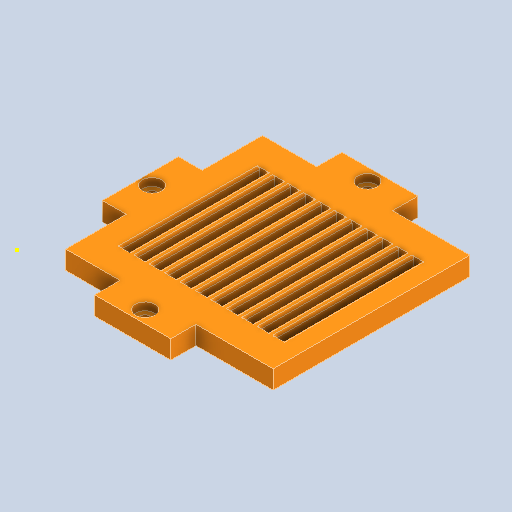
# Autodesk Inventor part: Tapa - Caja para Electrónica
Saved by Autodesk Inventor 2026 (Build 300175050, 175E)
## iProperties
Created: 2026-02-11
Part Number: Tapa - Caja para Electrónica
Material: Genérico
Document SubType Name: Modeling
Designer: bello
Density: 1 g/cm^3
Appearance: Naranja
Author: bello
Autodesk Inventor part; units mm, degrees
ref_plane "YZ Plane" through (0, 0, 0) normal (1, 0, 0) x (0, 1, 0)
ref_plane "XZ Plane" through (0, 0, 0) normal (0, 1, 0) x (-1, 0, 0)
ref_plane "XY Plane" through (0, 0, 0) normal (0, 0, 1) x (1, 0, 0)
sketch "Boceto1" plane through (0, 0, 0) normal (0, 1, 0) x (-1, 0, 0)
  line L0 (0, 0) -> (-75, 0)
  line L1 (-75, 0) -> (-75, -80)
  line L2 (-75, -80) -> (0, -80)
  line L3 (0, -80) -> (0, 0)
  dimension "d0" = 80
  dimension "d1" = 75
  constraints: 8 end point, 2 parallel, 1 horizontal, 1 perpendicular
  measures "d0" distance of L2.end L0.start
  measures "d1" distance of L1.end L2.end
extrude "Extrusión1" add sketch "Boceto1" along normal blind 6
sketch "Boceto2" plane through (0, 6, 0) normal (0, 1, 0) x (1, 0, 0)
  line L0 (0, 0) -> (75, 0) projected
  line L1 (25, 0) -> (25, 8)
  line L2 (25, 8) -> (7.5, 8)
  line L3 (7.5, 8) -> (7.5, 27.5)
  line L4 (7.5, 27.5) -> (0, 27.5)
  line L5 (0, 27.5) -> (0, 40)
  line L6 (25, 0) -> (50, 0)
  line L7 (50, 0) -> (50, 8)
  line L8 (50, 8) -> (75, 8)
  line L9 (75, 0) -> (75, 80) projected
  line L10 (-21.9373, 40) -> (100.0778, 40)
  line L11 (25, 0) -> (50, 0)
  line L12 (25, 80) -> (25, 72)
  line L13 (25, 72) -> (7.5, 72)
  line L14 (7.5, 72) -> (7.5, 52.5)
  line L15 (7.5, 52.5) -> (0, 52.5)
  line L16 (0, 52.5) -> (0, 40)
  line L17 (50, 80) -> (50, 72)
  line L18 (50, 72) -> (75, 72)
  line L19 (25, 80) -> (50, 80)
  line L20 (75, 80) -> (0, 80) projected
  line L21 (0, 80) -> (0, 0) projected
  dimension "d4" = 12.5
  dimension "d7" = 8
  dimension "d8" = 25
  dimension "d9" = 25
  dimension "d10" = 12.5
  dimension "d11" = 27.5
  dimension "d12" = 27.5
  dimension "d13" = 8
  dimension "d14" = 8
  dimension "d15" = 8
  dimension "d16" = 7.5
  dimension "d17" = 25
  dimension "d18" = 25
  dimension "d19" = 25
  dimension "d20" = 25
  constraints: 36 end point, 8 symmetric about line, 4 perpendicular, 3 point on line, 2 horizontal, 1 collinear, 1 vertical
  measures "d4" distance of L4.end L5.end
  measures "d7" distance between parallel lines of L0 L2
  measures "d8" distance of L1.start L6.end
  measures "d9" distance of L7.end L8.end
  measures "d10" distance of L16.start L5.end
  measures "d11" distance between parallel lines of L20 L15
  measures "d12" distance between parallel lines of L0 L4
  measures "d13" distance between parallel lines of L20 L13
  measures "d14" distance between parallel lines of L20 L18
  measures "d15" distance between parallel lines of L0 L8
  measures "d16" distance between parallel lines of L21 L14
  measures "d17" distance of L12.start L19.end
  measures "d18" distance of L17.end L18.end
  measures "d19" distance between parallel lines of L21 L12
  measures "d20" distance between parallel lines of L21 L1
extrude "Extrusión2" cut sketch "Boceto2" against normal through all contours L21 L4 L3 L2 L1 L0 | L7 L8 L9 L0 | L21 L20 L12 L13 L14 L15 | L18 L17 L20 L9
sketch "Boceto3" plane through (0, 6, 0) normal (0, 1, 0) x (1, 0, 0)
  circle A0 centre (3.75, 40) radius 1.5
  circle A1 centre (37.5, 76) radius 1.5
  circle A2 centre (37.5, 4) radius 1.5
  line L0 (7.5, 52.5) -> (0, 52.5) projected
  line L1 (0, 52.5) -> (0, 27.5) projected
  line L2 (50, 80) -> (25, 80) projected
  line L3 (25, 0) -> (50, 0) projected
  line L4 (50, 0) -> (50, 8) projected
  line L5 (50, 72) -> (50, 80) projected
  point P0 (0, 0)
  dimension "d23" = 3
  dimension "d24" = 12.5
  dimension "d25" = 3.75
  dimension "d26" = 4
  dimension "d27" = 4
  dimension "d28" = 12.5
  dimension "d29" = 12.5
  constraints: 3 centre point, 2 equal radius
  measures "d23" diameter of A0
  measures "d24" distance from line of L0 A0.centre
  measures "d25" distance from line of L1 A0.centre
  measures "d26" distance from line of L2 A1.centre
  measures "d27" distance from line of L3 A2.centre
  measures "d28" distance from line of L4 A2.centre
  measures "d29" distance from line of L5 A1.centre
extrude "Extrusión3" cut sketch "Boceto3" against normal through all
sketch "Boceto4" plane through (0, 6, 0) normal (0, 1, 0) x (1, 0, 0)
  circle A0 centre (3.75, 40) radius 1.5 projected
  circle A1 centre (3.75, 40) radius 3.1
  circle A2 centre (37.5, 4) radius 1.5 projected
  circle A3 centre (37.5, 4) radius 3.1
  circle A4 centre (37.5, 76) radius 1.5 projected
  circle A5 centre (37.5, 76) radius 3.1
  point P0 (0, 0)
  dimension "d32" = 6.2
  constraints: 3 centre point, 3 coincident, 2 equal radius
  measures "d32" diameter of A1
extrude "Extrusión4" cut sketch "Boceto4" against normal blind 2.5 contours A0 | A1 | A2 | A3 | A5
sketch "Boceto5" plane through (0, 6, 0) normal (0, 1, 0) x (1, 0, 0)
  line L0 (0, 52.5) -> (0, 27.5) projected
  line L1 (7.5, 52.5) -> (0, 52.5) projected
  line L2 (0, 52.5) -> (7.5, 52.5)
  line L3 (7.5, 52.5) -> (7.5, 52.3)
  line L4 (7.5, 52.3) -> (0, 52.3)
  line L5 (0, 52.3) -> (0, 52.5)
  line L6 (25, 80) -> (25, 72) projected
  line L7 (25, 80) -> (25.2, 80)
  line L8 (25.2, 80) -> (25.2, 71.85)
  line L9 (25.2, 71.85) -> (25, 71.85)
  line L10 (25, 71.85) -> (25, 80)
  line L11 (7.5, 72) -> (25, 72)
  line L12 (25, 72) -> (25, 71.85)
  line L13 (25, 71.85) -> (7.5, 71.85)
  line L14 (7.5, 71.85) -> (7.5, 72)
  line L15 (7.5, 52.3) -> (7.65, 52.3)
  line L16 (7.65, 52.3) -> (7.65, 72)
  line L17 (7.65, 72) -> (7.5, 72)
  line L18 (7.5, 72) -> (7.5, 52.3)
  line L19 (50, 80) -> (25, 80) projected
  line L20 (50, 80) -> (49.8, 80)
  line L21 (49.8, 80) -> (49.8, 71.85)
  line L22 (49.8, 71.85) -> (50, 71.85)
  line L23 (50, 71.85) -> (50, 80)
  line L24 (50, 71.85) -> (75, 71.85)
  line L25 (75, 71.85) -> (75, 72)
  line L26 (75, 72) -> (50, 72)
  line L27 (50, 72) -> (50, 71.85)
  line L28 (50, 8) -> (75, 8) projected
  line L29 (75, 8) -> (74.8, 8)
  line L30 (74.8, 8) -> (74.8, 72)
  line L31 (74.8, 72) -> (75, 72)
  line L32 (75, 72) -> (75, 8)
  line L33 (-2.8758, 40) -> (82.3038, 40)
  line L34 (7.5, 27.5) -> (0, 27.5)
  line L35 (0, 27.5) -> (7.5, 27.5)
  line L36 (7.5, 27.5) -> (7.5, 27.7)
  line L37 (7.5, 27.7) -> (0, 27.7)
  line L38 (0, 27.7) -> (0, 27.5)
  line L39 (25, 0) -> (25, 8)
  line L40 (25, 0) -> (25.2, 0)
  line L41 (25.2, 0) -> (25.2, 8.15)
  line L42 (25.2, 8.15) -> (25, 8.15)
  line L43 (25, 8.15) -> (25, 0)
  line L44 (7.5, 8) -> (25, 8)
  line L45 (25, 8) -> (25, 8.15)
  line L46 (25, 8.15) -> (7.5, 8.15)
  line L47 (7.5, 8.15) -> (7.5, 8)
  line L48 (7.5, 27.7) -> (7.65, 27.7)
  line L49 (7.65, 27.7) -> (7.65, 8)
  line L50 (7.65, 8) -> (7.5, 8)
  line L51 (7.5, 8) -> (7.5, 27.7)
  line L52 (50, 0) -> (49.8, 0)
  line L53 (49.8, 0) -> (49.8, 8.15)
  line L54 (49.8, 8.15) -> (50, 8.15)
  line L55 (50, 8.15) -> (50, 0)
  line L56 (50, 8.15) -> (75, 8.15)
  line L57 (75, 8.15) -> (75, 8)
  line L58 (75, 8) -> (50, 8)
  line L59 (50, 8) -> (50, 8.15)
  point P0 (0, 0)
  point P1 (7.5, 8.15)
  point P2 (7.65, 8.15)
  point P3 (0, 27.7)
  point P4 (74.8, 71.85)
  point P5 (74.8, 8.15)
  point P6 (0, 52.3)
  point P7 (7.65, 71.85)
  point P8 (7.5, 71.85)
  dimension "d35" = 0.2
  dimension "d36" = 0.15
  dimension "d37" = 0.2
  dimension "d38" = 0.15
  dimension "d39" = 0.2
  dimension "d40" = 0.15
  dimension "d41" = 0.2
  constraints: 110 end point, 21 symmetric about line, 14 parallel, 10 horizontal, 7 perpendicular, 5 point on line
  measures "d35" distance between parallel lines of L1 L4
  measures "d36" distance of L3.end L15.end
  measures "d37" distance of L8.end L9.end
  measures "d38" distance of L11.end L9.end
  measures "d39" distance of L21.end L22.end
  measures "d40" distance of L26.end L22.end
  measures "d41" distance of L30.end L31.end
extrude "Extrusión5" cut sketch "Boceto5" against normal blind 6 contours L1 L3 L4 L0 | L37 L36 L34 L0 | L18 L13 L16 L15 L3 | L14 L11 L16 L13 | L33 L32 L56 L30 | L30 L24 L32 L33 | L16 L11 L10 L13 | L48 L49 L46 L51 L36 | L56 L32 L28 L30 | L30 L28 L55 L56 | L30 L26 L25 L24 | L24 L23 L26 L30 | L10 L6 L7 L8 L9 | L55 L52 L53 L54 | L22 L21 L19 L23 | L46 L49 L44 L47 | L46 L43 L44 L49 | L42 L41 L40 L39 L43
sketch "Boceto6" plane through (0, 6, 0) normal (0, 1, 0) x (1, 0, 0)
  point P0 (0, 0)
sketch "Boceto7" plane through (0, 6, 0) normal (0, 1, 0) x (1, 0, 0)
  line L0 (13.5, 17.5) -> (68.5, 17.5)
  line L1 (68.5, 17.5) -> (68.5, 62.5)
  line L2 (68.5, 62.5) -> (13.5, 62.5)
  line L3 (13.5, 62.5) -> (13.5, 17.5)
  line L4 (0, 52.3) -> (0, 27.7) projected
  line L5 (49.8, 80) -> (25.2, 80) projected
  line L6 (13.5, 17.5) -> (16, 17.5)
  line L7 (16, 17.5) -> (16, 62.5)
  line L8 (16, 62.5) -> (13.5, 62.5)
  line L9 (13.5, 62.5) -> (13.5, 17.5)
  line L10 (18.5, 17.5) -> (18.5, 62.5)
  line L11 (21, 17.5) -> (21, 62.5)
  line L12 (23.5, 17.5) -> (23.5, 62.5)
  line L13 (26, 17.5) -> (26, 62.5)
  line L14 (28.5, 17.5) -> (28.5, 62.5)
  line L15 (31, 17.5) -> (31, 62.5)
  line L16 (33.5, 17.5) -> (33.5, 62.5)
  line L17 (36, 17.5) -> (36, 62.5)
  line L18 (38.5, 17.5) -> (38.5, 62.5)
  line L19 (41, 17.5) -> (41, 62.5)
  line L20 (43.5, 17.5) -> (43.5, 62.5)
  line L21 (46, 17.5) -> (46, 62.5)
  line L22 (48.5, 17.5) -> (48.5, 62.5)
  line L23 (51, 17.5) -> (51, 62.5)
  line L24 (53.5, 17.5) -> (53.5, 62.5)
  line L25 (56, 17.5) -> (56, 62.5)
  line L26 (58.5, 17.5) -> (58.5, 62.5)
  line L27 (61, 17.5) -> (61, 62.5)
  line L28 (63.5, 17.5) -> (63.5, 62.5)
  line L29 (66, 17.5) -> (66, 62.5)
  point P0 (0, 0)
  point P1 (0, 40)
  point P2 (37.5, 80)
  dimension "d44" = 45
  dimension "d45" = 55
  dimension "d46" = 22.5
  dimension "d47" = 31
  dimension "d48" = 2.5
  dimension "d51" = 2.5
  constraints: 52 end point, 40 horizontal alignment, 23 parallel, 2 midpoint, 1 horizontal, 1 perpendicular, 1 vertical, 7 other
  measures "d44" distance of L3.start L3.end
  measures "d45" distance of L1.end L3.start
  measures "d46" vertical distance of point (0, 40) L3.end
  measures "d47" horizontal distance of point (37.5, 80) L1.end
  measures "d48" distance of L8.end L7.end
  measures "d51" distance of L6.end L10.start
extrude "Extrusión6" cut sketch "Boceto7" against normal blind 6 contours L7 L2 L10 L0 | L11 L2 L12 L0 | L13 L2 L14 L0 | L15 L2 L16 L0 | L17 L2 L18 L0 | L19 L2 L20 L0 | L21 L2 L22 L0 | L23 L2 L24 L0 | L25 L2 L26 L0 | L27 L2 L28 L0 | L29 L2 L1 L0
fillet "Empalme1" radius 0.7 22 edges at (66, 6, -40) (63.5, 6, -40) (61, 6, -40) (58.5, 6, -40) (56, 6, -40) (53.5, 6, -40) (51, 6, -40) (48.5, 6, -40) (46, 6, -40) (43.5, 6, -40) (41, 6, -40) (38.5, 6, -40) (68.5, 6, -40) (36, 6, -40) (33.5, 6, -40) (31, 6, -40) (28.5, 6, -40) (26, 6, -40) (23.5, 6, -40) (21, 6, -40) (18.5, 6, -40) (16, 6, -40)
